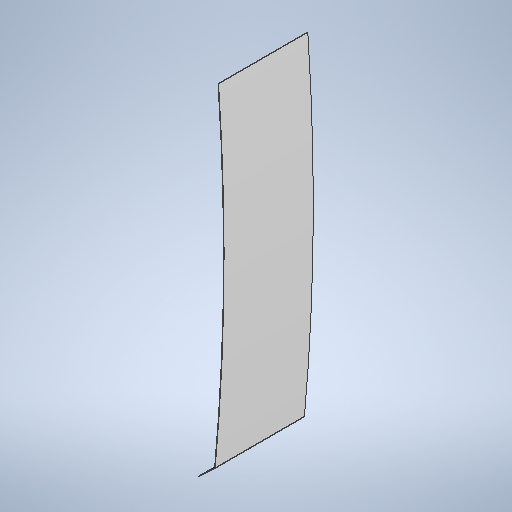
# Autodesk Inventor part: MSC 023 sheet left-right board hip
Saved by Autodesk Inventor 2025 (Build 290162010, 162A)
## iProperties
Created: 2024-04-18
Part Number: MSC 023 sheet left-right board hip
Material: Stainless Steel AISI 304
Document SubType Name: Sheet Metal
Designer: admin
Stock Number: МОО 023 лист левый-правый борт поясница
Mass: 48027.3 g
Surface Area: 40202.8 cm^2
Volume: 6003.41 cm^3
Density: 8 g/cm^3
Flat Pattern Width: 50 cm
Flat Pattern Length: 200.001 cm
Flat Pattern Area: 10000 cm^2
Sheet Metal Rule: AISI304 3mm Die 32
Sheet Metal Width: 500,000 mm
Sheet Metal Length: 2000,007 mm
Sheet Metal Area: 1000003,591 mm^2
Appearance: Default
Author: admin
Autodesk Inventor part; units mm, degrees
ref_plane "YZ Plane" through (0, 0, 0) normal (1, 0, 0) x (0, 1, 0)
ref_plane "XZ Plane" through (0, 0, 0) normal (0, 1, 0) x (-1, 0, 0)
ref_plane "XY Plane" through (0, 0, 0) normal (0, 0, 1) x (1, 0, 0)
sketch "Sketch1" plane through (0, 0, 0) normal (0, 0, 1) x (1, 0, 0)
  line L0 (-750, 0) -> (750, 0) construction
  line L1 (750, 0) -> (750, -2700) construction
  line L2 (750, -2700) -> (-750, -2700) construction
  line L3 (-750, -2700) -> (-750, 0) construction
  line L4 (800, 50) -> (-800, 50) construction
  line L5 (-800, 50) -> (-800, -2750) construction
  line L6 (-800, -2750) -> (800, -2750) construction
  line L7 (800, -2750) -> (800, 50) construction
  line L8 (-850, 100) -> (850, 100) construction
  line L9 (850, 100) -> (850, -2800) construction
  line L10 (850, -2800) -> (-850, -2800) construction
  line L11 (-850, -2800) -> (-850, 100) construction
  arc A0 (750, 0) -> (743.691501, 0.841272) centre (0, -5600) ccw construction
  line L12 (-750, -2100) -> (750, -2100) construction
  line L13 (115.485997, -2697.8227) -> (660.767125, -2184.072909) construction
  arc A1 (750, -2100) -> (750.178737, -2098.125829) centre (-10250, -1050) ccw construction
  line L14 (750, 0) -> (749.60177, -2.973451) construction
  arc A2 (750, -3.026786) -> (0, 47) centre (-0.2, -5602.999996) ccw construction
  line L15 (750, 0) -> (747.013575, -0.285068) construction
  arc A3 (768.074958, -251.105003) -> (747.4657, -5.032602) centre (-10252.989673, -1050.251043) ccw construction
  arc A4 (750.602724, -6.333527) -> (743.691501, 0.841272) centre (742.638487, -7.089123) ccw construction
  arc A5 (747.4657, -5.032602) -> (744.874766, -2.342571) centre (744.479151, -5.316372) ccw construction
  line L16 (750, -2100) -> (752.986425, -2100.285068) construction
  arc A6 (752.986425, -2100.285068) -> (772.222599, -225.731848) centre (-10246.98931, -1050.030895) ccw construction
  line L17 (750, -2100) -> (752.057249, -2102.183512) construction
  line L18 (752.05726, -2102.183502) -> (752.057249, -2102.183512) construction
  arc A7 (748.630029, -2101.290751) -> (750.178737, -2098.125829) centre (745.201281, -2097.651564) ccw
  line L19 (0, -2697) -> (110.793766, -2697) construction
  line L20 (112.851015, -2696.183512) -> (676.905813, -2164.745655) construction
  arc A8 (110, -2700) -> (115.485997, -2697.8227) centre (110, -2692) ccw construction
  arc A9 (110.793766, -2697) -> (112.851015, -2696.183512) centre (110.793766, -2694) ccw construction
  line L21 (676.905813, -2164.745655) -> (678.963062, -2166.929168) construction
  line L22 (752.05726, -2102.183502) -> (662.824374, -2186.256422) construction
  line L23 (662.824374, -2186.256422) -> (660.767125, -2184.072909) construction
  arc A10 (747.4657, -5.032602) -> (747.013575, -0.285068) centre (-10252.989673, -1050.251043) ccw construction
  arc A11 (743.691501, 0.841272) -> (0, 50) centre (0, -5600) ccw construction
  arc A12 (750.602724, -6.333527) -> (750, 0) centre (-10250, -1050) ccw construction
  line L24 (771.067103, -250.88805) -> (768.074958, -251.105003) construction
  line L25 (769.230952, -225.95557) -> (772.222599, -225.731848) construction
  arc A13 (769.230952, -225.95557) -> (750.602724, -6.333527) centre (-10250, -1050) ccw construction
  line L26 (0, 100) -> (0, 50) construction
  line L27 (0, -2700) -> (0, -2697) construction
  line L28 (0, 47) -> (0, 0) construction
  line L29 (0, 50) -> (0, 47) construction
  arc A14 (752.057249, -2102.183512) -> (752.986425, -2100.285068) centre (749.999823, -2099.999913) ccw construction
  line L30 (660.767125, -2184.072909) -> (748.630029, -2101.290751)
  arc A15 (750.178737, -2098.125829) -> (769.230952, -225.95557) centre (-10250, -1050) ccw
  line L31 (748.630029, -2101.290751) -> (750, -2100) construction
  point P0 (0, -2750)
  dimension "d54" = 1500
  dimension "d55" = 2700
  dimension "d58" = 2100
  dimension "d68" = 8
  dimension "d70" = 3
  dimension "d75" = 5
  dimension "d83" = 8
  dimension "d86" = 3
  dimension "d112" = 251.771
  dimension "d113" = 50
  dimension "d114" = 50
  dimension "d115" = 3
  dimension "d116" = 25
  dimension "d117" = 110
  dimension "d118" = 25
  dimension "d119" = 122.6
  measures "d54" distance of L0.start L0.end
  measures "d55" distance of L0.end L1.end
  measures "d58" distance between parallel lines of L12 L0
  measures "d68" radius of A4
  measures "d70" radius of A5
  measures "d75" radius of A7
  measures "d83" radius of A8
  measures "d86" radius of A9
  measures "d112" distance of L0.end L24.start
  measures "d113" distance between parallel lines of L4 L8
  measures "d114" distance between parallel lines of L0 L4
  measures "d115" distance of L26.end L28.start
  measures "d116" distance of L24.start L25.start
  measures "d117" distance from line of L27 A8.centre
  measures "d118" distance of L13.end L21.end
  measures "d119" distance of L12.end L13.end
contour flange "Contour Flange2" sketch "Sketch1" thickness 3 bend radius 5 width 500 along (0, 0, 1) mid plane no both sides no wall seen from (704.698577, -2142.68183, 0) lies toward (0.6857497, -0.7278375, 0) curves L30 A7 A15
bend "Bend2"
corner "Corner2"
sketch "Sketch2" plane through (750.687278, -2103.474264, 0) normal (0.6857497, -0.7278375, 0) x (0.7278375, 0.6857497, 0)
  line L0 (-120.717751, 0) -> (-120.717751, 500)
  line L1 (-120.717751, 500) -> (0, 500)
  line L2 (-70.717751, 475) -> (-58.717751, 475) construction
  line L3 (-58.717751, 475) -> (-58.717751, 315) construction
  line L4 (-58.717751, 315) -> (-70.717751, 315) construction
  line L5 (-70.717751, 315) -> (-70.717751, 475) construction
  point P0 (896.078441, 0)
  dimension "d120" = 12
  dimension "d121" = 160
  dimension "d122" = 25
  dimension "d123" = 50
  constraints: 2 other
  measures "d120" distance of L3.end L4.end
  measures "d121" distance between parallel lines of L2 L4
  measures "d122" distance between parallel lines of L1 L2
  measures "d123" distance between parallel lines of L0 L5
mark "Mark1"
equation "\"d36\" = Thickness"
equation "\"d37\" = BendReliefWidth"
equation "\"d38\" = BendReliefDepth"
equation "\"d39\" = MinimumRemnant"
equation "\"d40\" = TransitionRadius"
equation "\"d42\" = BendRadius"
equation "\"d44\" = CornerReliefSize"
equation "\"d45\" = GapSize"
equation "\"d46\" = JacobiRadiusSize"
equation "\"BendReliefWidth\" = Thickness"
equation "\"BendReliefDepth\" = 0.5 * Thickness"
equation "\"CornerReliefSize\" = 4 * Thickness"
equation "\"MinimumRemnant\" = 2 * Thickness"
equation "\"GapSize\" = Thickness"
equation "\"Thickness\" = 3"
equation "\"TransitionRadius\" = 5"
equation "\"BendRadius\" = 5"
equation "\"JacobiRadiusSize\" = 5"
body "Solid3"
